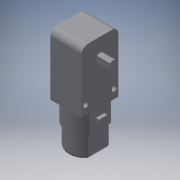
# Autodesk Inventor part: DCMotor
Saved by Autodesk Inventor 2017 (Build 210142000, 142)
## iProperties
Created: 2020-08-22
Part Number: DCMotor
Material: Generic
Document SubType Name: Modeling
Designer: agustin
Density: 1 g/cm^3
Appearance: Default
Author: agustin
Autodesk Inventor part; units mm, degrees
ref_plane "YZ Plane" through (0, 0, 0) normal (1, 0, 0) x (0, 1, 0)
ref_plane "XZ Plane" through (0, 0, 0) normal (0, 1, 0) x (-1, 0, 0)
ref_plane "XY Plane" through (0, 0, 0) normal (0, 0, 1) x (1, 0, 0)
sketch "Sketch1" plane through (0, 0, 0) normal (1, 0, 0) x (0, 1, 0)
  line L0 (0, 0) -> (33, 0)
  line L1 (37, -4) -> (37, -18.2)
  line L2 (33, -22.2) -> (0, -22.2)
  line L3 (0, -22.2) -> (0, 0)
  arc A0 (33, -22.2) -> (37, -18.2) centre (33, -18.2) ccw
  arc A1 (37, -4) -> (33, 0) centre (33, -4) ccw
  constraints: 8 end point, 4 point on circle, 2 centre point, 2 parallel, 1 horizontal, 1 perpendicular
extrude "Extrusion1" add sketch "Sketch1" along normal blind 19
sketch "Sketch2" plane through (19, 0, 0) normal (1, 0, 0) x (0, 0, -1)
  line L0 (0, 33) -> (0, 0) projected
  line L1 (22.2, 37) -> (0, 37)
  line L2 (0, 37) -> (0, 26)
  line L3 (22.2, 26) -> (22.2, 37)
  line L4 (0, 31.5) -> (0, 26)
  circle A0 centre (11.1, 26) radius 2.65
  dimension "d9" = 11
  dimension "d11" = 5.3
  constraints: 8 end point, 1 centre point, 1 horizontal, 1 parallel, 1 perpendicular, 1 point on line
  measures "d9" distance of L2.end L1.end
  measures "d11" diameter of A0
extrude "Extrusion2" add sketch "Sketch2" along normal blind 8
sketch "Sketch3" plane through (27, 26, -11.1) normal (1, 0, 0) x (0, 0, -1)
  line L0 (1.85, 0) -> (1.85, -3.8405)
  line L1 (1.85, -3.8405) -> (0, -3.8405)
  line L2 (1.85, -3.8405) -> (-1.85, -3.8405)
  line L3 (-1.85, -3.8405) -> (-1.85, 4.0175)
  line L4 (-1.85, 4.0175) -> (1.85, 4.0175)
  line L5 (1.85, 4.0175) -> (1.85, -3.8405)
  line L6 (1.85, 4.0175) -> (3.7589, 4.0175)
  line L7 (3.7589, 4.0175) -> (3.7589, -3.8405)
  line L8 (3.7589, -3.8405) -> (1.85, -3.8405)
  line L9 (1.85, -3.8405) -> (1.85, 4.0175)
  line L10 (-1.85, 4.0175) -> (-3.5435, 4.0175)
  line L11 (-3.5435, 4.0175) -> (-3.5435, -3.8405)
  line L12 (-3.5435, -3.8405) -> (-1.85, -3.8405)
  line L13 (-1.85, -3.8405) -> (-1.85, 4.0175)
  point P0 (-11.1, -26)
  dimension "d14" = 1.85
  dimension "d15" = 3.7
  constraints: 28 end point, 6 parallel, 3 horizontal, 3 perpendicular, 1 point on line
  measures "d14" distance of L0.end L1.end
  measures "d15" distance of L3.end L4.end
extrude "Extrusion3" cut sketch "Sketch3" against normal blind 8 contours L5 L6 L7 L8 L0 | L3 L12 L11 L10
sketch "Sketch4" plane through (19, 0, 0) normal (1, 0, 0) x (0, 0, -1)
  line L0 (0, 0) -> (22.2, 0) projected
  line L1 (0, 0) -> (22.2, 0)
  line L2 (22.2, 0) -> (22.2, 5.5)
  line L3 (0, 5.5) -> (0, 0)
  circle A0 centre (2.5, 5.5) radius 1.5
  circle A1 centre (19.7, 5.5) radius 1.5
  dimension "d18" = 5.5
  dimension "d20" = 3
  dimension "d22" = 3
  constraints: 6 end point, 2 centre point, 1 horizontal, 1 parallel, 1 perpendicular
  measures "d18" distance of L2.end L1.end
  measures "d20" diameter of A0
  measures "d22" diameter of A1
extrude "Extrusion4" cut sketch "Sketch4" against normal blind 20
sketch "Sketch5" plane through (0, 0, -22.2) normal (0, -1, 0) x (1, 0, 0)
  line L0 (0, 22.2) -> (19, 22.2) projected
  line L1 (0, 0) -> (19, 0) projected
  line L2 (19, 18.2) -> (19, 22.2) projected
  line L3 (19, 22.2) -> (10, 22.2)
  line L4 (18, 0) -> (19, 0)
  line L5 (19, 4.6031) -> (19, 17.5969)
  line L6 (0.8056, 17.3188) -> (0.8056, 4.8812)
  arc A0 (0.8056, 4.8812) -> (19, 4.6031) centre (10, 11.1) ccw
  arc A1 (19, 17.5969) -> (0.8056, 17.3188) centre (10, 11.1) ccw
  arc A2 (1.8056, 5.1956) -> (18, 4.9348) centre (10, 11.1) ccw
  arc A3 (18, 17.2652) -> (1.8056, 17.0044) centre (10, 11.1) ccw
  line L7 (1.8056, 17.0044) -> (1.8056, 5.1956)
  line L8 (0.8056, 4.8812) -> (0.8056, 17.3188)
  line L9 (18, 17.2652) -> (18, 4.9348)
  line L10 (19, 4.6031) -> (19, 17.5969)
  constraints: 16 end point, 8 point on circle, 4 centre point, 3 parallel, 1 coincident, 1 horizontal, 1 perpendicular, 1 point on line
extrude "Extrusion5" add sketch "Sketch5" along normal blind 11.5
sketch "Sketch6" plane through (18, 0, -17.2652) normal (0, -1, 0) x (1, 0, 0)
  line L0 (-16.1944, 12.0697) -> (-16.1944, 0.2608) projected
  arc A0 (-16.1944, 0.2608) -> (0, 0) centre (-8, 6.1652) ccw projected
  line L1 (0, 0) -> (0, 12.3305) projected
  arc A1 (0, 12.3305) -> (-16.1944, 12.0697) centre (-8, 6.1652) ccw projected
  line L2 (-16.1944, 12.0697) -> (-16.1944, 0.2608) projected
  arc A2 (-16.1944, 0.2608) -> (0, 0) centre (-8, 6.1652) ccw projected
  line L3 (0, 0) -> (0, 12.3305) projected
  arc A3 (0, 12.3305) -> (-16.1944, 12.0697) centre (-8, 6.1652) ccw projected
  point P0 (-18, 17.2652)
extrude "Extrusion6" add sketch "Sketch6" along normal blind 25
fillet "Fillet1" radius 2 4 edges at (18, -25, -11.1) (9.8374, -25, -21.1987) (1.8056, -25, -11.1) (9.8374, -25, -1.0013)
sketch "Sketch7" plane through (19, 0, 0) normal (1, 0, 0) x (0, 0, -1)
  line L0 (4.6031, 0) -> (4.6031, -11.5) projected
  line L1 (17.5969, 0) -> (17.5969, -11.5) projected
  line L2 (22.2, 0) -> (0, 0) projected
  line L3 (13.6, -4.25) -> (8.6, -4.25)
  line L4 (8.6, -4.25) -> (8.6, -7.25)
  line L5 (8.6, -7.25) -> (13.6, -7.25)
  line L6 (13.6, -7.25) -> (13.6, -4.25)
  line L7 (13.6, -4.25) -> (8.6, -7.25) construction
  line L8 (8.6, -4.25) -> (13.6, -7.25) construction
  dimension "d33" = 5
  dimension "d34" = 3
  constraints: 12 end point, 2 parallel, 1 horizontal, 1 perpendicular
  measures "d33" distance of L5.end L4.end
  measures "d34" distance of L4.end L3.end
extrude "Extrusion7" add sketch "Sketch7" along normal blind 2
sketch "Sketch8" plane through (0.8056, 0, -17.3188) normal (-1, 0, 0) x (0, 0, 1)
  line L0 (-4.8812, 0) -> (17.3188, 0) projected
  line L1 (3.7188, -4.25) -> (3.7188, -7.25) projected
  line L2 (8.7188, -7.25) -> (3.7188, -7.25)
  line L3 (3.7188, -7.25) -> (3.7188, -4.25)
  line L4 (3.7188, -4.25) -> (8.7188, -4.25)
  line L5 (8.7188, -4.25) -> (8.7188, -7.25)
  line L6 (8.7188, -7.25) -> (3.7188, -4.25) construction
  line L7 (3.7188, -7.25) -> (8.7188, -4.25) construction
  point P0 (6.2188, -5.75)
  constraints: 12 end point, 2 midpoint, 2 parallel, 1 horizontal, 1 perpendicular
extrude "Extrusion8" add sketch "Sketch8" along normal blind 2
scale "Scale1" factors (2, 2, 2) then translate (-19, -12.75, 11.1) bodies 1
scale "Scale2" factors (0.5, 0.5, 0.5) then translate (9.5, 6.375, -5.55) bodies 1
body "Solid1"
